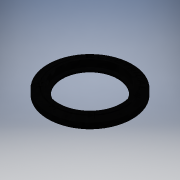
# Autodesk Inventor part: Team Pin Electrical
Saved by Autodesk Inventor 2016 (Build 200138000, 138)
## iProperties
Created: 2016-02-20
Part Number: Team Pin Electrical
Material: Generic
Document SubType Name: Modeling
Designer: RoksBot
Density: 1 g/cm^3
Appearance: Black
Author: RoksBot
Autodesk Inventor part; units mm, degrees
ref_plane "YZ Plane" through (0, 0, 0) normal (1, 0, 0) x (0, 1, 0)
ref_plane "XZ Plane" through (0, 0, 0) normal (0, 1, 0) x (-1, 0, 0)
ref_plane "XY Plane" through (0, 0, 0) normal (0, 0, 1) x (1, 0, 0)
sketch "Sketch1" plane through (0, 0, 0) normal (0, 0, 1) x (1, 0, 0)
  line L0 (0, 0) -> (0, 8.664595) construction
  line L1 (20.9931, 1.27) -> (20.9931, 5.715)
  line L2 (20.9931, 5.715) -> (27.9781, 3.81)
  line L3 (27.9781, 3.81) -> (27.9781, 0)
  line L4 (27.9781, 0) -> (20.9931, 0)
  line L5 (20.9931, 1.27) -> (18.4531, 1.27)
  line L6 (18.4531, 1.27) -> (18.4531, 0)
  line L7 (18.4531, 0) -> (20.9931, 0)
  dimension "d0" = 20.9931
  dimension "d1" = 4.445
  dimension "d2" = 1.27
  dimension "d3" = 2.54
  dimension "d4" = 3.81
  dimension "d5" = 6.985
  constraints: 16 end point, 2 parallel, 2 perpendicular, 2 vertical, 1 horizontal, 1 horizontal alignment
  measures "d0" distance between parallel lines of L0 L1
  measures "d1" distance from line of L5 L1.end
  measures "d2" distance of L5.end L6.end
  measures "d3" distance between parallel lines of L1 L6
  measures "d4" distance of L2.end L3.end
  measures "d5" distance between parallel lines of L1 L3
revolve "Revolution1" add sketch "Sketch1" angle 360 about axis through (0, 0, 0) along (0, 1, 0)
sketch "Sketch2" plane through (0, 1.27, 0) normal (0, 1, 0) x (1, 0, 0)
  circle A0 centre (0, 0) radius 18.4531
  circle A1 centre (0, 0) radius 18.4531
  circle A2 centre (0, 0) radius 20.9931
  circle A3 centre (0, 0) radius 27.9781
  circle A4 centre (0, 0) radius 23.5331 construction
  circle A5 centre (-20.32, 11.870316) radius 0.635
  line L0 (-20.634692, 12.421854) -> (-23.44965, 14.066265)
  line L1 (-23.44965, 14.066265) -> (-23.76995, 13.517965)
  line L2 (-23.76995, 13.517965) -> (-20.954992, 11.873554)
  line L3 (-18.1268, 10.589116) -> (-24.1581, 14.112415) construction
  arc A6 (-20.867836, 11.549223) -> (-21.272578, -10.785571) centre (0, 0) ccw
  arc A7 (-20.315793, 11.23533) -> (-20.709525, -10.491886) centre (0, 0) ccw
  circle A8 centre (-20.736735, -11.126302) radius 0.635
  arc A9 (-20.749114, -11.761182) -> (-18.917348, -14.525325) centre (0, 0) ccw
  arc A10 (-20.193077, -11.454419) -> (-18.421715, -14.128145) centre (0, 0) ccw
  line L4 (-17.33162, -13.254588) -> (-16.812519, -16.644068)
  line L5 (-16.812519, -16.644068) -> (-20.007445, -15.398883)
  line L6 (-20.007445, -15.398883) -> (-17.33162, -13.254588)
  line L7 (-17.75334, -18.211739) -> (-15.077515, -16.067445)
  line L8 (-15.077515, -16.067445) -> (-15.474606, -15.571921)
  line L9 (-15.474606, -15.571921) -> (-18.150432, -17.716216)
  line L10 (-18.150432, -17.716216) -> (-17.75334, -18.211739)
  line L11 (-17.75334, -18.211739) -> (-15.474606, -15.571921) construction
  line L12 (-15.077515, -16.067445) -> (-18.150432, -17.716216) construction
  arc A11 (-16.008472, -16.813474) -> (-10.00022, -20.951365) centre (0, 0) ccw
  arc A12 (-16.508379, -17.214079) -> (-10.266961, -21.527671) centre (0, 0) ccw
  circle A13 centre (-9.634539, -21.470502) radius 0.635
  arc A14 (-9.003627, -21.39857) -> (-2.111155, -23.11941) centre (0, 0) ccw
  arc A15 (-9.256828, -21.980952) -> (-2.155415, -23.753006) centre (0, 0) ccw
  line L13 (-2.013809, -21.725877) -> (0.829097, -23.643147)
  line L14 (0.829097, -23.643147) -> (-2.252761, -25.146541)
  line L15 (-2.252761, -25.146541) -> (-2.013809, -21.725877)
  line L16 (1.343077, -25.39773) -> (1.582029, -21.977066)
  line L17 (1.582029, -21.977066) -> (0.948573, -21.932815)
  line L18 (0.948573, -21.932815) -> (0.709621, -25.353479)
  line L19 (0.709621, -25.353479) -> (1.343077, -25.39773)
  line L20 (1.343077, -25.39773) -> (0.948573, -21.932815) construction
  line L21 (1.582029, -21.977066) -> (0.709621, -25.353479) construction
  arc A16 (1.498894, -23.167162) -> (8.614533, -21.558152) centre (0, 0) ccw
  arc A17 (1.454252, -23.806223) -> (8.857144, -22.145025) centre (0, 0) ccw
  circle A18 centre (9.244039, -21.6415) radius 0.635
  arc A19 (9.619063, -21.129073) -> (15.558144, -17.231025) centre (0, 0) ccw
  arc A20 (9.875321, -21.710116) -> (15.993742, -17.693256) centre (0, 0) ccw
  line L22 (14.600088, -16.214394) -> (17.937106, -15.4255)
  line L23 (17.937106, -15.4255) -> (16.9518, -18.709889)
  line L24 (16.9518, -18.709889) -> (14.600088, -16.214394)
  line L25 (19.57509, -16.237745) -> (17.223379, -13.74225)
  line L26 (17.223379, -13.74225) -> (16.76125, -14.177752)
  line L27 (16.76125, -14.177752) -> (19.112962, -16.673247)
  line L28 (19.112962, -16.673247) -> (19.57509, -16.237745)
  line L29 (19.57509, -16.237745) -> (16.76125, -14.177752) construction
  line L30 (17.223379, -13.74225) -> (19.112962, -16.673247) construction
  arc A21 (18.041572, -14.610468) -> (19.892926, -11.968107) centre (0, 0) ccw
  arc A22 (18.480927, -15.076685) -> (20.440919, -12.289017) centre (0, 0) ccw
  circle A23 centre (20.444814, -11.654029) radius 0.635
  line L31 (19.327699, 11.717344) -> (21.022058, 12.588074)
  line L32 (21.022058, 12.588074) -> (21.312301, 12.023287)
  line L33 (21.312301, 12.023287) -> (19.617942, 11.152557)
  line L34 (19.617942, 11.152557) -> (19.327699, 11.717344)
  line L35 (19.327699, 11.717344) -> (21.312301, 12.023287) construction
  line L36 (21.022058, 12.588074) -> (19.617942, 11.152557) construction
  line L37 (19.946537, 9.893538) -> (22.205683, 11.054511)
  line L38 (22.205683, 11.054511) -> (21.91544, 11.619297)
  line L39 (21.91544, 11.619297) -> (19.656294, 10.458324)
  line L40 (19.656294, 10.458324) -> (19.946537, 9.893538)
  line L41 (19.946537, 9.893538) -> (21.91544, 11.619297) construction
  line L42 (22.205683, 11.054511) -> (19.656294, 10.458324) construction
  line L43 (20.101171, 8.545119) -> (23.151019, 10.112433)
  line L44 (23.151019, 10.112433) -> (22.860775, 10.67722)
  line L45 (22.860775, 10.67722) -> (19.810928, 9.109906)
  line L46 (19.810928, 9.109906) -> (20.101171, 8.545119)
  line L47 (20.101171, 8.545119) -> (22.860775, 10.67722) construction
  line L48 (23.151019, 10.112433) -> (19.810928, 9.109906) construction
  line L49 (0, 0) -> (29.254796, 15.034015) construction
  arc A24 (20.989212, -11.327141) -> (21.891947, 9.465398) centre (0, 0) ccw
  arc A25 (20.433869, -11.019123) -> (21.325871, 9.174492) centre (0, 0) ccw
  line L50 (-21.651868, 14.781039) -> (-22.669258, 13.904548)
  line L51 (-22.669258, 13.904548) -> (-22.956293, 14.072225)
  line L52 (-22.956293, 14.072225) -> (-22.692483, 15.388934)
  line L53 (-22.692483, 15.388934) -> (-22.407225, 15.222295)
  line L54 (-22.407225, 15.222295) -> (-22.602684, 14.338846)
  line L55 (-22.602684, 14.338846) -> (-21.930017, 14.943525)
  line L56 (-21.930017, 14.943525) -> (-21.651868, 14.781039)
  spline S0 degree 2 poles (-21.790026, 13.36113) (-21.892222, 13.42083) (-22.031845, 13.571524) (-22.063792, 13.661702) knots 0 0 0 1 2 2 2
  spline S1 degree 2 poles (-22.063792, 13.661702) (-22.093443, 13.751729) (-22.067758, 13.954845) (-22.003387, 14.065038) knots 0 0 0 1 2 2 2
  spline S2 degree 2 poles (-22.003387, 14.065038) (-21.933824, 14.184118) (-21.762101, 14.30669) (-21.666082, 14.322113) knots 0 0 0 1 2 2 2
  spline S3 degree 2 poles (-21.666082, 14.322113) (-21.574655, 14.337835) (-21.378517, 14.290004) (-21.287874, 14.237054) knots 0 0 0 1 2 2 2
  spline S4 degree 2 poles (-21.287874, 14.237054) (-21.219448, 14.197081) (-21.101283, 14.085144) (-21.052214, 14.009995) knots 0 0 0 1 2 2 2
  line L57 (-21.052214, 14.009995) -> (-21.180957, 13.789609)
  line L58 (-21.180957, 13.789609) -> (-21.213837, 13.808816)
  spline S5 degree 2 poles (-21.213837, 13.808816) (-21.221008, 13.833268) (-21.244676, 13.89477) (-21.263029, 13.924562) knots 0 0 0 1 2 2 2
  spline S6 degree 2 poles (-21.263029, 13.924562) (-21.282122, 13.95717) (-21.339867, 14.019509) (-21.383411, 14.044946) knots 0 0 0 1 2 2 2
  spline S7 degree 2 poles (-21.383411, 14.044946) (-21.482052, 14.102569) (-21.670932, 14.02816) (-21.739456, 13.910858) knots 0 0 0 1 2 2 2
  spline S8 degree 2 poles (-21.739456, 13.910858) (-21.812134, 13.786446) (-21.768248, 13.596326) (-21.672273, 13.54026) knots 0 0 0 1 2 2 2
  spline S9 degree 2 poles (-21.672273, 13.54026) (-21.623397, 13.511708) (-21.537549, 13.491356) (-21.501545, 13.491778) knots 0 0 0 1 2 2 2
  spline S10 degree 2 poles (-21.501545, 13.491778) (-21.466949, 13.491831) (-21.409899, 13.503797) (-21.388782, 13.50934) knots 0 0 0 1 2 2 2
  line L59 (-21.388782, 13.50934) -> (-21.355902, 13.490132)
  line L60 (-21.355902, 13.490132) -> (-21.485164, 13.268857)
  spline S11 degree 2 poles (-21.485164, 13.268857) (-21.513091, 13.27206) (-21.585389, 13.280921) (-21.620275, 13.290573) knots 0 0 0 1 2 2 2
  spline S12 degree 2 poles (-21.620275, 13.290573) (-21.663828, 13.301712) (-21.735818, 13.329464) (-21.790026, 13.36113) knots 0 0 0 1 2 2 2
  spline S13 degree 2 poles (-20.99468, 12.896514) (-21.096875, 12.956213) (-21.236499, 13.106908) (-21.268446, 13.197085) knots 0 0 0 1 2 2 2
  spline S14 degree 2 poles (-21.268446, 13.197085) (-21.298097, 13.287113) (-21.272412, 13.490228) (-21.208041, 13.600421) knots 0 0 0 1 2 2 2
  spline S15 degree 2 poles (-21.208041, 13.600421) (-21.138478, 13.719501) (-20.966755, 13.842073) (-20.870735, 13.857496) knots 0 0 0 1 2 2 2
  spline S16 degree 2 poles (-20.870735, 13.857496) (-20.779309, 13.873219) (-20.583171, 13.825388) (-20.492528, 13.772437) knots 0 0 0 1 2 2 2
  spline S17 degree 2 poles (-20.492528, 13.772437) (-20.424102, 13.732465) (-20.305937, 13.620528) (-20.256868, 13.545378) knots 0 0 0 1 2 2 2
  line L61 (-20.256868, 13.545378) -> (-20.385611, 13.324992)
  line L62 (-20.385611, 13.324992) -> (-20.418491, 13.3442)
  spline S18 degree 2 poles (-20.418491, 13.3442) (-20.425662, 13.368651) (-20.44933, 13.430153) (-20.467683, 13.459946) knots 0 0 0 1 2 2 2
  spline S19 degree 2 poles (-20.467683, 13.459946) (-20.486776, 13.492553) (-20.544521, 13.554892) (-20.588065, 13.580329) knots 0 0 0 1 2 2 2
  spline S20 degree 2 poles (-20.588065, 13.580329) (-20.686706, 13.637952) (-20.875586, 13.563544) (-20.94411, 13.446241) knots 0 0 0 1 2 2 2
  spline S21 degree 2 poles (-20.94411, 13.446241) (-21.016788, 13.32183) (-20.972902, 13.131709) (-20.876927, 13.075644) knots 0 0 0 1 2 2 2
  spline S22 degree 2 poles (-20.876927, 13.075644) (-20.828051, 13.047092) (-20.742203, 13.02674) (-20.706199, 13.027162) knots 0 0 0 1 2 2 2
  spline S23 degree 2 poles (-20.706199, 13.027162) (-20.671603, 13.027214) (-20.614553, 13.03918) (-20.593436, 13.044723) knots 0 0 0 1 2 2 2
  line L63 (-20.593436, 13.044723) -> (-20.560556, 13.025515)
  line L64 (-20.560556, 13.025515) -> (-20.689818, 12.80424)
  spline S24 degree 2 poles (-20.689818, 12.80424) (-20.717745, 12.807443) (-20.790043, 12.816304) (-20.824929, 12.825956) knots 0 0 0 1 2 2 2
  spline S25 degree 2 poles (-20.824929, 12.825956) (-20.868482, 12.837096) (-20.940472, 12.864847) (-20.99468, 12.896514) knots 0 0 0 1 2 2 2
  point P0 (-18.050528, -15.09918)
  point P1 (-18.669533, -14.326736)
  point P2 (-16.613973, -16.89183)
  point P3 (-1.145825, -23.505188)
  point P4 (-2.133285, -23.436209)
  point P5 (1.145825, -23.665272)
  point P6 (16.496331, -16.783261)
  point P7 (15.775944, -17.462142)
  point P8 (18.16817, -15.207749)
  point P9 (20.32, 11.870316)
  point P10 (20.930988, 10.756418)
  point P11 (21.480973, 9.61117)
  point P12 (20.930988, 10.756418)
  dimension "d7" = 2.54
  dimension "d18" = 1.27
  dimension "d21" = 0.635
  dimension "d22" = 3.175
  dimension "d23" = 20.32
  dimension "d24" = 0.635
  dimension "d25" = 0.3175
  dimension "d26" = 1.27
  dimension "d27" = 0.635
  dimension "d28" = 0.3175
  dimension "d29" = 3.429
  dimension "d30" = 3.429
  dimension "d31" = 0.635
  dimension "d32" = 0.635
  dimension "d33" = 0.3175
  dimension "d34" = 3.81
  dimension "d35" = 1.27
  dimension "d36" = 7.62
  dimension "d37" = 0.635
  dimension "d38" = 0.3175
  dimension "d39" = 3.429
  dimension "d40" = 7.62
  dimension "d42" = 0.635
  dimension "d43" = 3.429
  dimension "d44" = 1.14582
  dimension "d45" = 1.14582
  dimension "d46" = 0.635
  dimension "d47" = 0.3175
  dimension "d48" = 1.27
  dimension "d49" = 7.62
  dimension "d50" = 0.635
  dimension "d51" = 0.3175
  dimension "d52" = 7.62
  dimension "d53" = 3.429
  dimension "d54" = 0.635
  dimension "d55" = 3.429
  dimension "d56" = 1.27
  dimension "d57" = 0.635
  dimension "d58" = 0.3175
  dimension "d59" = 3.81
  dimension "d60" = 3.429
  dimension "d61" = 2.54
  dimension "d62" = 1.905
  dimension "d63" = 0.635
  dimension "d64" = 0.635
  dimension "d65" = 0.635
  dimension "d66" = 20.32
  dimension "d67" = 0.635
  dimension "d68" = 0.3175
  constraints: 100 end point, 52 point on circle, 21 centre point, 21 parallel, 19 midpoint, 16 point on line, 8 perpendicular, 1 coincident, 1 concentric, 59 other
  measures "d18" diameter of A5
  measures "d21" distance between parallel lines of L2 L0
  measures "d22" distance edge to line of A5 L1
  measures "d23" horizontal distance of A5.centre point (0, 0)
  measures "d24" radial gap between concentric circles of A7 A6
  measures "d26" diameter of A8
  measures "d27" radial gap between concentric circles of A9 A10
  measures "d29" distance of L5.end L4.start
  measures "d30" distance of L8.end L9.end
  measures "d31" distance of L7.end L8.end
  measures "d32" radial gap between concentric circles of A12 A11
  measures "d34" distance of point (-18.67, -14.327) A8.centre
  measures "d35" diameter of A13
  measures "d36" distance from line of L7 A13.centre
  measures "d37" radial gap between concentric circles of A15 A14
  measures "d39" distance of L14.end L13.start
  measures "d40" distance from line of L15 A13.centre
  measures "d42" distance of L16.end L17.end
  measures "d43" distance of L17.end L18.end
  measures "d44" horizontal distance of point (0, 0) point (-1.146, -23.505)
  measures "d45" horizontal distance of A0.centre point (1.146, -23.665)
  measures "d46" radial gap between concentric circles of A17 A16
  measures "d48" diameter of A18
  measures "d49" distance from line of A18.centre L16
  measures "d50" radial gap between concentric circles of A20 A19
  measures "d52" distance from line of L24 A18.centre
  measures "d53" distance of L23.end L22.start
  measures "d54" distance between parallel lines of L27 L25
  measures "d55" distance of L26.end L27.end
  measures "d56" diameter of A23
  measures "d57" radial gap between concentric circles of A22 A21
  measures "d59" distance of A21.start A23.centre
  measures "d60" distance of L43.start L43.end
  measures "d61" distance of L37.start L37.end
  measures "d62" distance of L32.end L33.end
  measures "d63" distance of L31.end L32.end
  measures "d64" distance between parallel lines of L45 L37
  measures "d65" distance between parallel lines of L39 L33
  measures "d66" horizontal distance of point (0, 0) point (20.32, 11.87)
  measures "d67" radial gap between concentric circles of A25 A24
extrude "Extrusion1" cut sketch "Sketch2" along normal through all contours A5 | L27 L26 L25 L28 | L18 L17 L16 L19 | L9 L8 L7 L10 | A5 L2 L1 L0 | A7 A8 A6 A5 | A8 | A8 A10 L6 A9 | L6 L4 L5 | A11 A13 A12 L7 | A13 | A14 L15 A15 A13 | L15 L13 L14 | A16 A18 A17 L16 | A18 | A19 L24 A20 A18 | L24 L22 L23 | A21 A23 A22 L25 | A23 | A25 L43 A24 A23 | L43 L46 L45 L44 | L31 L32 L33 L34 | L40 L39 L38 L37 | L50 L51 L52 L53 L54 L55 L56 | S0 S1 S2 S3 S4 L57 L58 S5 S6 S7 S8 S9 S10 L59 L60 S11 S12 | S13 S14 S15 S16 S17 L61 L62 S18 S19 S20 S21 S22 S23 L63 L64 S24 S25
sketch "Sketch3" plane through (0, 1.27, 0) normal (0, 1, 0) x (1, 0, 0)
  circle A0 centre (0, 0) radius 18.4531
  circle A1 centre (0, 0) radius 20.9931
  circle A2 centre (0, 0) radius 20.9931
  circle A3 centre (0, 0) radius 27.9781
  circle A4 centre (0, 0) radius 22.8981
  line L0 (-17.473523, 14.891403) -> (-20.277521, 17.655017)
  line L1 (-20.277521, 17.655017) -> (-17.612894, 20.358582)
  line L2 (-17.612894, 20.358582) -> (-17.146014, 19.898426)
  line L3 (-17.146014, 19.898426) -> (-19.259523, 17.754032)
  line L4 (-19.259523, 17.754032) -> (-18.616205, 17.119979)
  line L5 (-18.616205, 17.119979) -> (-17.324021, 18.431045)
  line L6 (-17.324021, 18.431045) -> (-16.859855, 17.973564)
  line L7 (-16.859855, 17.973564) -> (-18.152038, 16.662498)
  line L8 (-18.152038, 16.662498) -> (-17.397429, 15.918757)
  line L9 (-17.397429, 15.918757) -> (-15.262517, 18.084866)
  line L10 (-15.262517, 18.084866) -> (-14.787493, 17.616684)
  line L11 (-14.787493, 17.616684) -> (-17.473523, 14.891403)
  line L12 (-13.814282, 18.306781) -> (-15.628338, 21.01375)
  line L13 (-15.628338, 21.01375) -> (-15.014125, 21.425361)
  line L14 (-15.014125, 21.425361) -> (-13.543785, 19.231291)
  line L15 (-13.543785, 19.231291) -> (-11.536512, 20.576451)
  line L16 (-11.536512, 20.576451) -> (-11.192796, 20.063552)
  line L17 (-11.192796, 20.063552) -> (-13.814282, 18.306781)
  line L18 (-10.428399, 20.437492) -> (-11.7223, 23.428195)
  line L19 (-11.7223, 23.428195) -> (-8.710609, 24.731175)
  line L20 (-8.710609, 24.731175) -> (-8.468476, 24.171512)
  line L21 (-8.468476, 24.171512) -> (-10.801574, 23.162118)
  line L22 (-10.801574, 23.162118) -> (-10.542794, 22.563978)
  line L23 (-10.542794, 22.563978) -> (-9.136639, 23.172338)
  line L24 (-9.136639, 23.172338) -> (-8.894505, 22.612674)
  line L25 (-8.894505, 22.612674) -> (-10.30066, 22.004314)
  line L26 (-10.30066, 22.004314) -> (-9.988914, 21.283747)
  line L27 (-9.988914, 21.283747) -> (-7.627832, 22.305247)
  line L28 (-7.627832, 22.305247) -> (-7.388726, 21.752579)
  line L29 (-7.388726, 21.752579) -> (-10.428399, 20.437492)
  line L30 (-4.332703, 25.200647) -> (-6.306951, 24.773391)
  line L31 (-6.306951, 24.773391) -> (-5.877276, 22.787967)
  line L32 (-5.877276, 22.787967) -> (-3.903028, 23.215224)
  line L33 (-3.903028, 23.215224) -> (-4.061032, 23.945324)
  line L34 (-4.061032, 23.945324) -> (-3.310974, 23.975066)
  line L35 (-3.310974, 23.975066) -> (-3.221492, 23.561591)
  spline S0 degree 2 poles (-3.221492, 23.561591) (-3.123948, 23.110867) (-3.403658, 22.691583) (-3.869282, 22.590815) knots 0 0 0 1 2 2 2
  line L36 (-3.869282, 22.590815) -> (-5.657281, 22.203865)
  spline S1 degree 2 poles (-5.657281, 22.203865) (-6.122905, 22.103097) (-6.541077, 22.35965) (-6.641039, 22.82155) knots 0 0 0 1 2 2 2
  line L37 (-6.641039, 22.82155) -> (-6.987681, 24.423299)
  spline S2 degree 2 poles (-6.987681, 24.423299) (-7.085225, 24.874023) (-6.808434, 25.288776) (-6.346535, 25.388738) knots 0 0 0 1 2 2 2
  line L38 (-6.346535, 25.388738) -> (-4.558536, 25.775687)
  spline S3 degree 2 poles (-4.558536, 25.775687) (-4.096637, 25.875649) (-3.664066, 25.606614) (-3.568134, 25.16334) knots 0 0 0 1 2 2 2
  line L39 (-3.568134, 25.16334) -> (-3.49155, 24.809465)
  line L40 (-3.49155, 24.809465) -> (-4.191628, 24.548773)
  line L41 (-4.191628, 24.548773) -> (-4.332703, 25.200647)
  line L42 (-0.289949, 25.548393) -> (-0.218409, 22.900555)
  line L43 (-0.218409, 22.900555) -> (-0.953708, 22.880689)
  line L44 (-0.953708, 22.880689) -> (-1.025248, 25.528527)
  line L45 (-1.025248, 25.528527) -> (-2.492036, 25.488897)
  line L46 (-2.492036, 25.488897) -> (-2.508506, 26.098471)
  line L47 (-2.508506, 26.098471) -> (1.167989, 26.197804)
  line L48 (1.167989, 26.197804) -> (1.184459, 25.588229)
  line L49 (1.184459, 25.588229) -> (-0.289949, 25.548393)
  line L50 (2.060505, 22.85946) -> (2.574924, 26.0772)
  line L51 (2.574924, 26.0772) -> (5.119009, 25.670479)
  spline S4 degree 2 poles (5.119009, 25.670479) (5.49159, 25.610914) (5.786685, 25.235669) (5.731332, 24.889433) knots 0 0 0 1 2 2 2
  line L52 (5.731332, 24.889433) -> (5.62183, 24.204487)
  spline S5 degree 2 poles (5.62183, 24.204487) (5.566478, 23.858251) (5.169702, 23.597474) (4.797121, 23.657039) knots 0 0 0 1 2 2 2
  line L53 (4.797121, 23.657039) -> (4.465939, 23.709985)
  line L54 (4.465939, 23.709985) -> (5.628246, 22.289087)
  line L55 (5.628246, 22.289087) -> (4.747601, 22.429875)
  line L56 (4.747601, 22.429875) -> (3.713251, 23.830316)
  line L57 (3.713251, 23.830316) -> (2.983144, 23.947038)
  line L58 (2.983144, 23.947038) -> (2.790613, 22.742738)
  line L59 (2.790613, 22.742738) -> (2.060505, 22.85946)
  line L60 (4.771797, 25.116166) -> (3.209969, 25.365855)
  line L61 (3.209969, 25.365855) -> (3.075197, 24.522845)
  line L62 (3.075197, 24.522845) -> (4.637025, 24.273156)
  spline S6 degree 2 poles (4.637025, 24.273156) (4.798853, 24.247285) (4.903013, 24.319404) (4.927681, 24.473705) knots 0 0 0 1 2 2 2
  line L63 (4.927681, 24.473705) -> (4.986042, 24.838759)
  spline S7 degree 2 poles (4.986042, 24.838759) (5.008304, 24.978006) (4.926098, 25.091498) (4.771797, 25.116166) knots 0 0 0 1 2 2 2
  line L64 (7.23196, 21.730143) -> (6.529876, 21.949546)
  line L65 (6.529876, 21.949546) -> (7.49957, 25.052537)
  line L66 (7.49957, 25.052537) -> (8.201654, 24.833134)
  line L67 (8.201654, 24.833134) -> (7.23196, 21.730143)
  line L68 (12.049617, 22.553307) -> (10.22885, 23.427956)
  line L69 (10.22885, 23.427956) -> (9.34925, 21.596883)
  line L70 (9.34925, 21.596883) -> (11.170017, 20.722234)
  line L71 (11.170017, 20.722234) -> (11.493472, 21.395574)
  line L72 (11.493472, 21.395574) -> (12.103832, 20.958616)
  line L73 (12.103832, 20.958616) -> (11.920651, 20.577285)
  spline S8 degree 2 poles (11.920651, 20.577285) (11.720967, 20.161601) (11.242777, 20.00232) (10.813351, 20.208605) knots 0 0 0 1 2 2 2
  line L74 (10.813351, 20.208605) -> (9.164354, 21.00074)
  spline S9 degree 2 poles (9.164354, 21.00074) (8.734928, 21.207025) (8.56231, 21.666253) (8.766945, 22.092243) knots 0 0 0 1 2 2 2
  line L75 (8.766945, 22.092243) -> (9.476566, 23.56947)
  spline S10 degree 2 poles (9.476566, 23.56947) (9.67625, 23.985154) (10.149354, 24.14265) (10.575345, 23.938015) knots 0 0 0 1 2 2 2
  line L76 (10.575345, 23.938015) -> (12.224342, 23.14588)
  spline S11 degree 2 poles (12.224342, 23.14588) (12.650332, 22.941245) (12.826656, 22.463325) (12.630272, 22.054511) knots 0 0 0 1 2 2 2
  line L77 (12.630272, 22.054511) -> (12.473495, 21.728148)
  line L78 (12.473495, 21.728148) -> (11.760818, 21.952111)
  line L79 (11.760818, 21.952111) -> (12.049617, 22.553307)
  line L80 (12.164059, 19.517431) -> (15.593119, 21.002927)
  line L81 (15.593119, 21.002927) -> (16.090539, 20.624443)
  line L82 (16.090539, 20.624443) -> (15.609602, 16.895733)
  line L83 (15.609602, 16.895733) -> (15.006025, 17.354992)
  line L84 (15.006025, 17.354992) -> (15.125318, 18.178934)
  line L85 (15.125318, 18.178934) -> (13.484439, 19.427472)
  line L86 (13.484439, 19.427472) -> (12.728206, 19.088174)
  line L87 (12.728206, 19.088174) -> (12.164059, 19.517431)
  line L88 (14.065873, 19.732156) -> (15.260894, 18.82287)
  line L89 (15.260894, 18.82287) -> (15.468092, 20.341387)
  line L90 (15.468092, 20.341387) -> (14.065873, 19.732156)
  line L91 (16.192597, 16.241073) -> (18.618953, 18.416223)
  line L92 (18.618953, 18.416223) -> (19.112496, 17.865681)
  line L93 (19.112496, 17.865681) -> (17.14587, 16.102665)
  line L94 (17.14587, 16.102665) -> (18.758788, 14.303472)
  line L95 (18.758788, 14.303472) -> (18.299058, 13.891338)
  line L96 (18.299058, 13.891338) -> (16.192597, 16.241073)
  dimension "d71" = 1.905
  constraints: 1 centre point, 1 coincident, 1 other
  measures "d71" radial gap between concentric circles of A1 A4
extrude "Extrusion2" cut sketch "Sketch3" along normal through all contours L65 L66 L67 L64 | L17 L12 L13 L14 L15 L16 | L11 L0 L1 L2 L3 L4 L5 L6 L7 L8 L9 L10 | L29 L18 L19 L20 L21 L22 L23 L24 L25 L26 L27 L28 | L36 S1 L37 S2 L38 S3 L39 L40 L41 L30 L31 L32 L33 L34 L35 S0 | L43 L44 L45 L46 L47 L48 L49 L42 | L74 S9 L75 S10 L76 S11 L77 L78 L79 L68 L69 L70 L71 L72 L73 S8 | L96 L91 L92 L93 L94 L95 | L50 L51 S4 L52 S5 L53 L54 L55 L56 L57 L58 L59 | L80 L81 L82 L83 L84 L85 L86 L87
equation "\"d25\" = 0.5 * d24"
equation "\"d26\" = d18"
equation "\"d30\" = d29"
equation "\"d33\" = 0.5 * d32"
equation "\"d35\" = d26"
equation "\"d38\" = 0.5 * d37"
equation "\"d39\" = d29"
equation "\"d40\" = d36"
equation "\"d42\" = d31"
equation "\"d43\" = d30"
equation "\"d44\" = d45"
equation "\"d47\" = 0.5 * d46"
equation "\"d48\" = d35"
equation "\"d49\" = d40"
equation "\"d51\" = 0.5 * d50"
equation "\"d52\" = d49"
equation "\"d53\" = d39"
equation "\"d54\" = d42"
equation "\"d55\" = d53"
equation "\"d56\" = d48"
equation "\"d58\" = 0.5 * d57"
equation "\"d59\" = d34"
equation "\"d65\" = d64"
body "Solid1"
